Autodesk Fusion 360 part; units mm, degrees
(part 5 of 11)
  spline S19 degree 5 poles (23.435, -47.1498) (23.4194, -47.1502) (23.3882, -47.1511) (23.3415, -47.1525) (23.2792, -47.1547) (23.2015, -47.1578) (23.1239, -47.1612) (23.0464, -47.1651) (22.9691, -47.1693) (22.8919, -47.1739) (22.8149, -47.179) (22.738, -47.1844) (22.6613, -47.1902) (22.5846, -47.1964) (22.5082, -47.2031) (22.4319, -47.2101) (22.3558, -47.2175) (22.2798, -47.2253) (22.204, -47.2336) (22.1283, -47.2422) (22.0528, -47.2512) (21.9775, -47.2607) (21.9023, -47.2706) (21.8274, -47.2809) (21.7526, -47.2916) (21.6779, -47.3027) (21.6035, -47.3143) (21.5293, -47.3262) (21.4552, -47.3386) (21.3814, -47.3515) (21.3077, -47.3647) (21.2343, -47.3784) (21.161, -47.3926) (21.088, -47.4072) (21.0152, -47.4222) (20.9426, -47.4377) (20.8702, -47.4536) (20.7981, -47.47) (20.7261, -47.4868) (20.6545, -47.5041) (20.583, -47.5219) (20.5118, -47.5401) (20.4409, -47.5588) (20.3702, -47.5781) (20.2998, -47.5978) (20.2296, -47.6179) (20.1598, -47.6386) (20.0902, -47.6598) (20.0208, -47.6814) (19.9518, -47.7036) (19.8831, -47.7263) (19.8147, -47.7496) (19.7466, -47.7734) (19.679, -47.7979) (19.6116, -47.8229) (19.5446, -47.8485) (19.4779, -47.8745) (19.4115, -47.9011) (19.3455, -47.9282) (19.2798, -47.956) (19.2147, -47.9844) (19.15, -48.0138) (19.086, -48.044) (19.0226, -48.0751) (18.9598, -48.107) (18.8973, -48.1395) (18.8351, -48.1724) (18.7733, -48.2058) (18.7119, -48.2397) (18.6513, -48.2748) (18.5921, -48.3117) (18.5461, -48.3432) (18.5126, -48.3682) (18.4908, -48.3855) (18.48, -48.3944) knots -1 -1 -1 -1 -1 -1 -0.98571429 -0.97142857 -0.95714286 -0.94285714 -0.92857143 -0.91428571 -0.9 -0.88571429 -0.87142857 -0.85714286 -0.84285714 -0.82857143 -0.81428571 -0.8 -0.78571429 -0.77142857 -0.75714286 -0.74285714 -0.72857143 -0.71428571 -0.7 -0.68571429 -0.67142857 -0.65714286 -0.64285714 -0.62857143 -0.61428571 -0.6 -0.58571429 -0.57142857 -0.55714286 -0.54285714 -0.52857143 -0.51428571 -0.5 -0.48571429 -0.47142857 -0.45714286 -0.44285714 -0.42857143 -0.41428571 -0.4 -0.38571429 -0.37142857 -0.35714286 -0.34285714 -0.32857143 -0.31428571 -0.3 -0.28571429 -0.27142857 -0.25714286 -0.24285714 -0.22857143 -0.21428571 -0.2 -0.18571429 -0.17142857 -0.15714286 -0.14285714 -0.12857143 -0.11428571 -0.1 -0.08571429 -0.07142857 -0.05714286 -0.04285714 -0.02857143 -0.01428571 0 0 0 0 0 0
  line L19 (18.48, -48.3944) -> (17.8629, -48.8983)
  arc A39 (15.7015, -48.7555) -> (17.8629, -48.8983) centre (16.8587, -47.6688) ccw
  arc A40 (15.7015, -48.7555) -> (14.881, -47.9278) centre (0, -63.5) ccw
  arc A41 (14.757, -45.7652) -> (14.881, -47.9278) centre (15.9777, -46.7801) ccw
  line L20 (14.757, -45.7652) -> (15.2663, -45.1525)
  spline S20 degree 5 poles (15.2663, -45.1525) (15.2753, -45.1418) (15.2928, -45.1201) (15.3181, -45.0869) (15.35, -45.0412) (15.3874, -44.9822) (15.423, -44.922) (15.4575, -44.8609) (15.4914, -44.7993) (15.5248, -44.7375) (15.5579, -44.6753) (15.5903, -44.6127) (15.622, -44.5496) (15.6528, -44.4858) (15.6826, -44.4215) (15.7117, -44.3565) (15.74, -44.2911) (15.7677, -44.2253) (15.7948, -44.1592) (15.8215, -44.0927) (15.8476, -44.0259) (15.8733, -43.9588) (15.8983, -43.8913) (15.9227, -43.8235) (15.9466, -43.7553) (15.9699, -43.6868) (15.9927, -43.618) (16.0149, -43.5488) (16.0367, -43.4794) (16.058, -43.4097) (16.0788, -43.3398) (16.0991, -43.2695) (16.1189, -43.199) (16.1383, -43.1282) (16.1571, -43.0572) (16.1755, -42.9859) (16.1934, -42.9144) (16.2109, -42.8426) (16.2279, -42.7706) (16.2445, -42.6984) (16.2606, -42.6259) (16.2762, -42.5532) (16.2915, -42.4803) (16.3062, -42.4072) (16.3206, -42.3339) (16.3345, -42.2604) (16.348, -42.1866) (16.361, -42.1127) (16.3736, -42.0385) (16.3858, -41.9642) (16.3976, -41.8897) (16.409, -41.815) (16.4199, -41.7401) (16.4305, -41.6651) (16.4406, -41.5898) (16.4503, -41.5144) (16.4596, -41.4388) (16.4685, -41.3631) (16.477, -41.2872) (16.4851, -41.2111) (16.4927, -41.1349) (16.5, -41.0585) (16.5069, -40.9819) (16.5134, -40.9052) (16.5195, -40.8284) (16.5252, -40.7514) (16.5305, -40.6743) (16.5354, -40.597) (16.54, -40.5196) (16.5441, -40.442) (16.5478, -40.3643) (16.5505, -40.3021) (16.5524, -40.2553) (16.5535, -40.2241) (16.5541, -40.2085) knots 0 0 0 0 0 0 0.01428571 0.02857143 0.04285714 0.05714286 0.07142857 0.08571429 0.1 0.11428571 0.12857143 0.14285714 0.15714286 0.17142857 0.18571429 0.2 0.21428571 0.22857143 0.24285714 0.25714286 0.27142857 0.28571429 0.3 0.31428571 0.32857143 0.34285714 0.35714286 0.37142857 0.38571429 0.4 0.41428571 0.42857143 0.44285714 0.45714286 0.47142857 0.48571429 0.5 0.51428571 0.52857143 0.54285714 0.55714286 0.57142857 0.58571429 0.6 0.61428571 0.62857143 0.64285714 0.65714286 0.67142857 0.68571429 0.7 0.71428571 0.72857143 0.74285714 0.75714286 0.77142857 0.78571429 0.8 0.81428571 0.82857143 0.84285714 0.85714286 0.87142857 0.88571429 0.9 0.91428571 0.92857143 0.94285714 0.95714286 0.97142857 0.98571429 1 1 1 1 1 1
  arc A42 (16.5541, -40.2085) -> (15.3942, -39.4262) centre (0, -63.5) ccw
  spline S21 degree 5 poles (15.3942, -39.4262) (15.3799, -39.4325) (15.3514, -39.4453) (15.3088, -39.4645) (15.2521, -39.4903) (15.1815, -39.5229) (15.1111, -39.5558) (15.041, -39.589) (14.9712, -39.6225) (14.9017, -39.6563) (14.8324, -39.6905) (14.7635, -39.7249) (14.6948, -39.7596) (14.6264, -39.7947) (14.5583, -39.8301) (14.4905, -39.8658) (14.423, -39.9017) (14.3558, -39.9381) (14.2889, -39.9747) (14.2223, -40.0116) (14.156, -40.0489) (14.09, -40.0864) (14.0244, -40.1243) (13.9591, -40.1625) (13.8941, -40.201) (13.8294, -40.2399) (13.765, -40.279) (13.701, -40.3185) (13.6374, -40.3583) (13.574, -40.3984) (13.5111, -40.4389) (13.4485, -40.4796) (13.3862, -40.5207) (13.3243, -40.5621) (13.2628, -40.6039) (13.2016, -40.646) (13.1409, -40.6884) (13.0805, -40.7311) (13.0205, -40.7742) (12.9609, -40.8176) (12.9017, -40.8614) (12.8429, -40.9055) (12.7845, -40.9499) (12.7265, -40.9947) (12.669, -41.0398) (12.612, -41.0853) (12.5553, -41.1312) (12.4991, -41.1774) (12.4433, -41.2239) (12.388, -41.2708) (12.3332, -41.3181) (12.279, -41.3658) (12.2252, -41.4138) (12.172, -41.4623) (12.1194, -41.5112) (12.0673, -41.5605) (12.0156, -41.6101) (11.9645, -41.66) (11.9139, -41.7104) (11.8638, -41.7611) (11.8145, -41.8124) (11.766, -41.8642) (11.7184, -41.9166) (11.6718, -41.9696) (11.6259, -42.0231) (11.5806, -42.0771) (11.5358, -42.1313) (11.4914, -42.1858) (11.4477, -42.2406) (11.4052, -42.2962) (11.3645, -42.3529) (11.3341, -42.3996) (11.3128, -42.4356) (11.2992, -42.4599) (11.2926, -42.4722) knots -1 -1 -1 -1 -1 -1 -0.98571429 -0.97142857 -0.95714286 -0.94285714 -0.92857143 -0.91428571 -0.9 -0.88571429 -0.87142857 -0.85714286 -0.84285714 -0.82857143 -0.81428571 -0.8 -0.78571429 -0.77142857 -0.75714286 -0.74285714 -0.72857143 -0.71428571 -0.7 -0.68571429 -0.67142857 -0.65714286 -0.64285714 -0.62857143 -0.61428571 -0.6 -0.58571429 -0.57142857 -0.55714286 -0.54285714 -0.52857143 -0.51428571 -0.5 -0.48571429 -0.47142857 -0.45714286 -0.44285714 -0.42857143 -0.41428571 -0.4 -0.38571429 -0.37142857 -0.35714286 -0.34285714 -0.32857143 -0.31428571 -0.3 -0.28571429 -0.27142857 -0.25714286 -0.24285714 -0.22857143 -0.21428571 -0.2 -0.18571429 -0.17142857 -0.15714286 -0.14285714 -0.12857143 -0.11428571 -0.1 -0.08571429 -0.07142857 -0.05714286 -0.04285714 -0.02857143 -0.01428571 0 0 0 0 0 0
  line L21 (11.2926, -42.4722) -> (10.9153, -43.174)
  arc A43 (8.8638, -43.8692) -> (10.9153, -43.174) centre (9.5171, -42.4223) ccw
  arc A44 (8.8638, -43.8692) -> (7.789, -43.4184) centre (0, -63.5) ccw
  arc A45 (6.8469, -41.4679) -> (7.789, -43.4184) centre (8.3631, -41.9384) ccw
  line L22 (6.8469, -41.4679) -> (7.083, -40.707)
  spline S22 degree 5 poles (7.083, -40.707) (7.0871, -40.6936) (7.095, -40.6669) (7.1057, -40.6265) (7.1177, -40.5721) (7.1297, -40.5033) (7.1395, -40.434) (7.148, -40.3644) (7.1557, -40.2946) (7.163, -40.2246) (7.1697, -40.1545) (7.1757, -40.0843) (7.1808, -40.0138) (7.1849, -39.9431) (7.1878, -39.8722) (7.1898, -39.8012) (7.1909, -39.7299) (7.1913, -39.6585) (7.1911, -39.587) (7.1903, -39.5154) (7.1889, -39.4437) (7.1869, -39.3719) (7.1842, -39.3) (7.1808, -39.2279) (7.1768, -39.1558) (7.1721, -39.0836) (7.1668, -39.0113) (7.1609, -38.9389) (7.1544, -38.8664) (7.1474, -38.7939) (7.1399, -38.7213) (7.1318, -38.6486) (7.1231, -38.5759) (7.1139, -38.5031) (7.1041, -38.4303) (7.0938, -38.3574) (7.083, -38.2844) (7.0717, -38.2114) (7.0598, -38.1384) (7.0475, -38.0653) (7.0346, -37.9922) (7.0213, -37.9191) (7.0075, -37.8459) (6.9931, -37.7727) (6.9783, -37.6994) (6.963, -37.6262) (6.9473, -37.5529) (6.931, -37.4796) (6.9143, -37.4063) (6.8972, -37.3329) (6.8795, -37.2596) (6.8614, -37.1862) (6.8429, -37.1129) (6.8239, -37.0395) (6.8045, -36.9661) (6.7846, -36.8927) (6.7642, -36.8193) (6.7435, -36.746) (6.7223, -36.6726) (6.7006, -36.5992) (6.6785, -36.5258) (6.656, -36.4525) (6.6331, -36.3791) (6.6098, -36.3058) (6.586, -36.2324) (6.5618, -36.1591) (6.5372, -36.0858) (6.5121, -36.0125) (6.4867, -35.9393) (6.4608, -35.8661) (6.4346, -35.7929) (6.4132, -35.7343) (6.3971, -35.6904) (6.3862, -35.6611) (6.3807, -35.6465) knots 0 0 0 0 0 0 0.01428571 0.02857143 0.04285714 0.05714286 0.07142857 0.08571429 0.1 0.11428571 0.12857143 0.14285714 0.15714286 0.17142857 0.18571429 0.2 0.21428571 0.22857143 0.24285714 0.25714286 0.27142857 0.28571429 0.3 0.31428571 0.32857143 0.34285714 0.35714286 0.37142857 0.38571429 0.4 0.41428571 0.42857143 0.44285714 0.45714286 0.47142857 0.48571429 0.5 0.51428571 0.52857143 0.54285714 0.55714286 0.57142857 0.58571429 0.6 0.61428571 0.62857143 0.64285714 0.65714286 0.67142857 0.68571429 0.7 0.71428571 0.72857143 0.74285714 0.75714286 0.77142857 0.78571429 0.8 0.81428571 0.82857143 0.84285714 0.85714286 0.87142857 0.88571429 0.9 0.91428571 0.92857143 0.94285714 0.95714286 0.97142857 0.98571429 1 1 1 1 1 1
  arc A46 (6.3807, -35.6465) -> (5.0097, -35.3676) centre (0, -63.5) ccw
  spline S23 degree 5 poles (5.0097, -35.3676) (4.999, -35.3789) (4.9776, -35.4016) (4.9455, -35.4357) (4.903, -35.4812) (4.8502, -35.5384) (4.7978, -35.5957) (4.7457, -35.6532) (4.6941, -35.7108) (4.6428, -35.7687) (4.5919, -35.8267) (4.5413, -35.8849) (4.4912, -35.9433) (4.4414, -36.0019) (4.392, -36.0606) (4.343, -36.1195) (4.2944, -36.1786) (4.2462, -36.2379) (4.1984, -36.2973) (4.1511, -36.3569) (4.1041, -36.4167) (4.0575, -36.4767) (4.0114, -36.5368) (3.9656, -36.5971) (3.9203, -36.6575) (3.8754, -36.7182) (3.831, -36.779) (3.7869, -36.8399) (3.7433, -36.9011) (3.7002, -36.9624) (3.6575, -37.0238) (3.6152, -37.0854) (3.5735, -37.1472) (3.5321, -37.2092) (3.4913, -37.2713) (3.4509, -37.3336) (3.411, -37.396) (3.3715, -37.4586) (3.3326, -37.5214) (3.2941, -37.5843) (3.2561, -37.6474) (3.2187, -37.7106) (3.1818, -37.774) (3.1454, -37.8376) (3.1095, -37.9013) (3.0742, -37.9652) (3.0394, -38.0292) (3.0052, -38.0934) (2.9715, -38.1577) (2.9383, -38.2222) (2.9058, -38.2869) (2.8739, -38.3517) (2.8426, -38.4167) (2.812, -38.4818) (2.7821, -38.5471) (2.7528, -38.6126) (2.7241, -38.6782) (2.696, -38.7439) (2.6684, -38.8098) (2.6416, -38.8758) (2.6157, -38.942) (2.5907, -39.0084) (2.5668, -39.0751) (2.544, -39.1419) (2.5221, -39.2089) (2.5009, -39.2761) (2.4802, -39.3433) (2.4601, -39.4106) (2.4407, -39.478) (2.4226, -39.5457) (2.4068, -39.6136) (2.3966, -39.6684) (2.3906, -39.7098) (2.3874, -39.7375) (2.386, -39.7514) knots -1 -1 -1 -1 -1 -1 -0.98571429 -0.97142857 -0.95714286 -0.94285714 -0.92857143 -0.91428571 -0.9 -0.88571429 -0.87142857 -0.85714286 -0.84285714 -0.82857143 -0.81428571 -0.8 -0.78571429 -0.77142857 -0.75714286 -0.74285714 -0.72857143 -0.71428571 -0.7 -0.68571429 -0.67142857 -0.65714286 -0.64285714 -0.62857143 -0.61428571 -0.6 -0.58571429 -0.57142857 -0.55714286 -0.54285714 -0.52857143 -0.51428571 -0.5 -0.48571429 -0.47142857 -0.45714286 -0.44285714 -0.42857143 -0.41428571 -0.4 -0.38571429 -0.37142857 -0.35714286 -0.34285714 -0.32857143 -0.31428571 -0.3 -0.28571429 -0.27142857 -0.25714286 -0.24285714 -0.22857143 -0.21428571 -0.2 -0.18571429 -0.17142857 -0.15714286 -0.14285714 -0.12857143 -0.11428571 -0.1 -0.08571429 -0.07142857 -0.05714286 -0.04285714 -0.02857143 -0.01428571 0 0 0 0 0 0
  line L23 (2.386, -39.7514) -> (2.306, -40.5441)
  arc A47 (0.6767, -41.9714) -> (2.306, -40.5441) centre (0.7266, -40.3847) ccw
  arc A48 (0.6767, -41.9714) -> (-0.4888, -41.9663) centre (0, -63.5) ccw
  arc A49 (-2.1056, -40.5248) -> (-0.4888, -41.9663) centre (-0.5248, -40.3793) ccw
  line L24 (-2.1056, -40.5248) -> (-2.1787, -39.7315)
  spline S24 degree 5 poles (-2.1787, -39.7315) (-2.18, -39.7176) (-2.1829, -39.6898) (-2.1885, -39.6484) (-2.1983, -39.5936) (-2.2135, -39.5254) (-2.231, -39.4577) (-2.2498, -39.3901) (-2.2693, -39.3226) (-2.2894, -39.2552) (-2.31, -39.1878) (-2.3313, -39.1206) (-2.3535, -39.0536) (-2.3769, -38.9868) (-2.4013, -38.9201) (-2.4266, -38.8537) (-2.4529, -38.7874) (-2.4798, -38.7213) (-2.5074, -38.6553) (-2.5355, -38.5895) (-2.5643, -38.5238) (-2.5936, -38.4582) (-2.6236, -38.3928) (-2.6543, -38.3276) (-2.6856, -38.2625) (-2.7176, -38.1975) (-2.7502, -38.1328) (-2.7833, -38.0681) (-2.817, -38.0036) (-2.8513, -37.9393) (-2.886, -37.8751) (-2.9213, -37.8111) (-2.9572, -37.7472) (-2.9935, -37.6835) (-3.0304, -37.6199) (-3.0678, -37.5565) (-3.1057, -37.4933) (-3.1441, -37.4302) (-3.183, -37.3672) (-3.2224, -37.3045) (-3.2622, -37.2418) (-3.3026, -37.1794) (-3.3433, -37.117) (-3.3846, -37.0549) (-3.4263, -36.9929) (-3.4685, -36.9311) (-3.5111, -36.8694) (-3.5541, -36.8079) (-3.5976, -36.7465) (-3.6416, -36.6854) (-3.6859, -36.6243) (-3.7307, -36.5635) (-3.7759, -36.5028) (-3.8215, -36.4423) (-3.8676, -36.3819) (-3.914, -36.3217) (-3.9609, -36.2617) (-4.0082, -36.2019) (-4.0559, -36.1422) (-4.1039, -36.0827) (-4.1524, -36.0233) (-4.2013, -35.9642) (-4.2505, -35.9052) (-4.3002, -35.8464) (-4.3502, -35.7877) (-4.4006, -35.7292) (-4.4514, -35.6709) (-4.5026, -35.6128) (-4.5541, -35.5549) (-4.606, -35.4971) (-4.6583, -35.4395) (-4.7004, -35.3936) (-4.7322, -35.3592) (-4.7534, -35.3364) (-4.764, -35.3249) knots 0 0 0 0 0 0 0.01428571 0.02857143 0.04285714 0.05714286 0.07142857 0.08571429 0.1 0.11428571 0.12857143 0.14285714 0.15714286 0.17142857 0.18571429 0.2 0.21428571 0.22857143 0.24285714 0.25714286 0.27142857 0.28571429 0.3 0.31428571 0.32857143 0.34285714 0.35714286 0.37142857 0.38571429 0.4 0.41428571 0.42857143 0.44285714 0.45714286 0.47142857 0.48571429 0.5 0.51428571 0.52857143 0.54285714 0.55714286 0.57142857 0.58571429 0.6 0.61428571 0.62857143 0.64285714 0.65714286 0.67142857 0.68571429 0.7 0.71428571 0.72857143 0.74285714 0.75714286 0.77142857 0.78571429 0.8 0.81428571 0.82857143 0.84285714 0.85714286 0.87142857 0.88571429 0.9 0.91428571 0.92857143 0.94285714 0.95714286 0.97142857 0.98571429 1 1 1 1 1 1
  arc A50 (-4.764, -35.3249) -> (-6.1374, -35.5919) centre (0, -63.5) ccw
  spline S25 degree 5 poles (-6.1374, -35.5919) (-6.143, -35.6065) (-6.1541, -35.6356) (-6.1707, -35.6794) (-6.1925, -35.7378) (-6.2194, -35.8107) (-6.2459, -35.8837) (-6.272, -35.9568) (-6.2977, -36.0298) (-6.3229, -36.1029) (-6.3478, -36.176) (-6.3722, -36.2491) (-6.3962, -36.3222) (-6.4198, -36.3954) (-6.4429, -36.4686) (-6.4656, -36.5417) (-6.4879, -36.6149) (-6.5097, -36.6881) (-6.5312, -36.7613) (-6.5521, -36.8345) (-6.5727, -36.9077) (-6.5927, -36.9809) (-6.6124, -37.0542) (-6.6316, -37.1274) (-6.6503, -37.2006) (-6.6686, -37.2738) (-6.6864, -37.3469) (-6.7037, -37.4201) (-6.7206, -37.4933) (-6.737, -37.5664) (-6.7529, -37.6395) (-6.7684, -37.7126) (-6.7833, -37.7857) (-6.7978, -37.8588) (-6.8118, -37.9318) (-6.8253, -38.0048) (-6.8383, -38.0777) (-6.8507, -38.1507) (-6.8627, -38.2236) (-6.8742, -38.2964) (-6.8851, -38.3692) (-6.8955, -38.442) (-6.9053, -38.5147) (-6.9146, -38.5873) (-6.9234, -38.6599) (-6.9316, -38.7324) (-6.9392, -38.8049) (-6.9463, -38.8773) (-6.9528, -38.9497) (-6.9587, -39.0219) (-6.9641, -39.0941) (-6.9687, -39.1662) (-6.9727, -39.2382) (-6.9761, -39.3101) (-6.9787, -39.3819) (-6.9807, -39.4536) (-6.9822, -39.5251) (-6.983, -39.5966) (-6.9832, -39.668) (-6.9827, -39.7393) (-6.9814, -39.8104) (-6.979, -39.8813) (-6.9756, -39.952) (-6.9711, -40.0225) (-6.9657, -40.0928) (-6.9596, -40.163) (-6.9529, -40.233) (-6.9458, -40.3029) (-6.9379, -40.3726) (-6.9287, -40.442) (-6.9173, -40.5108) (-6.9058, -40.5654) (-6.8955, -40.6059) (-6.8878, -40.6327) (-6.8838, -40.646) knots -1 -1 -1 -1 -1 -1 -0.98571429 -0.97142857 -0.95714286 -0.94285714 -0.92857143 -0.91428571 -0.9 -0.88571429 -0.87142857 -0.85714286 -0.84285714 -0.82857143 -0.81428571 -0.8 -0.78571429 -0.77142857 -0.75714286 -0.74285714 -0.72857143 -0.71428571 -0.7 -0.68571429 -0.67142857 -0.65714286 -0.64285714 -0.62857143 -0.61428571 -0.6 -0.58571429 -0.57142857 -0.55714286 -0.54285714 -0.52857143 -0.51428571 -0.5 -0.48571429 -0.47142857 -0.45714286 -0.44285714 -0.42857143 -0.41428571 -0.4 -0.38571429 -0.37142857 -0.35714286 -0.34285714 -0.32857143 -0.31428571 -0.3 -0.28571429 -0.27142857 -0.25714286 -0.24285714 -0.22857143 -0.21428571 -0.2 -0.18571429 -0.17142857 -0.15714286 -0.14285714 -0.12857143 -0.11428571 -0.1 -0.08571429 -0.07142857 -0.05714286 -0.04285714 -0.02857143 -0.01428571 0 0 0 0 0 0
  line L25 (-6.8838, -40.646) -> (-6.6544, -41.409)
  arc A51 (-7.6135, -43.3512) -> (-6.6544, -41.409) centre (-8.1746, -41.8662) ccw
  arc A52 (-7.6135, -43.3512) -> (-8.6921, -43.7925) centre (0, -63.5) ccw
  arc A53 (-10.7376, -43.0795) -> (-8.6921, -43.7925) centre (-9.3328, -42.3401) ccw
  line L26 (-10.7376, -43.0795) -> (-11.1087, -42.3745)
  spline S26 degree 5 poles (-11.1087, -42.3745) (-11.1152, -42.3621) (-11.1285, -42.3376) (-11.1495, -42.3015) (-11.1795, -42.2546) (-11.2197, -42.1975) (-11.2617, -42.1415) (-11.305, -42.0863) (-11.3489, -42.0314) (-11.3932, -41.9768) (-11.438, -41.9225) (-11.4834, -41.8686) (-11.5296, -41.8151) (-11.5767, -41.7623) (-11.6248, -41.7101) (-11.6737, -41.6584) (-11.7233, -41.6072) (-11.7734, -41.5565) (-11.8242, -41.5061) (-11.8754, -41.456) (-11.9271, -41.4063) (-11.9793, -41.3569) (-12.032, -41.308) (-12.0853, -41.2595) (-12.1392, -41.2113) (-12.1936, -41.1636) (-12.2485, -41.1162) (-12.3038, -41.0692) (-12.3596, -41.0225) (-12.4159, -40.9761) (-12.4726, -40.9301) (-12.5297, -40.8845) (-12.5872, -40.8392) (-12.6452, -40.7942) (-12.7036, -40.7496) (-12.7624, -40.7054) (-12.8217, -40.6614) (-12.8813, -40.6178) (-12.9413, -40.5746) (-13.0017, -40.5316) (-13.0625, -40.489) (-13.1236, -40.4467) (-13.1852, -40.4048) (-13.2471, -40.3631) (-13.3093, -40.3218) (-13.3719, -40.2808) (-13.4349, -40.2402) (-13.4982, -40.1998) (-13.5619, -40.1598) (-13.6259, -40.1201) (-13.6902, -40.0807) (-13.7549, -40.0416) (-13.8199, -40.0028) (-13.8852, -39.9644) (-13.9508, -39.9262) (-14.0168, -39.8884) (-14.083, -39.8509) (-14.1496, -39.8137) (-14.2165, -39.7768) (-14.2837, -39.7402) (-14.3512, -39.7039) (-14.419, -39.668) (-14.4871, -39.6323) (-14.5554, -39.597) (-14.6241, -39.5619) (-14.693, -39.5272) (-14.7623, -39.4928) (-14.8318, -39.4587) (-14.9016, -39.4248) (-14.9716, -39.3913) (-15.042, -39.3582) (-15.0985, -39.3318) (-15.141, -39.3122) (-15.1693, -39.2992) (-15.1835, -39.2928) knots 0 0 0 0 0 0 0.01428571 0.02857143 0.04285714 0.05714286 0.07142857 0.08571429 0.1 0.11428571 0.12857143 0.14285714 0.15714286 0.17142857 0.18571429 0.2 0.21428571 0.22857143 0.24285714 0.25714286 0.27142857 0.28571429 0.3 0.31428571 0.32857143 0.34285714 0.35714286 0.37142857 0.38571429 0.4 0.41428571 0.42857143 0.44285714 0.45714286 0.47142857 0.48571429 0.5 0.51428571 0.52857143 0.54285714 0.55714286 0.57142857 0.58571429 0.6 0.61428571 0.62857143 0.64285714 0.65714286 0.67142857 0.68571429 0.7 0.71428571 0.72857143 0.74285714 0.75714286 0.77142857 0.78571429 0.8 0.81428571 0.82857143 0.84285714 0.85714286 0.87142857 0.88571429 0.9 0.91428571 0.92857143 0.94285714 0.95714286 0.97142857 0.98571429 1 1 1 1 1 1
  arc A54 (-15.1835, -39.2928) -> (-16.3502, -40.065) centre (0, -63.5) ccw
  spline S27 degree 5 poles (-16.3502, -40.065) (-16.3498, -40.0806) (-16.3489, -40.1118) (-16.3475, -40.1585) (-16.3453, -40.2208) (-16.3422, -40.2985) (-16.3388, -40.3761) (-16.3349, -40.4536) (-16.3307, -40.5309) (-16.3261, -40.6081) (-16.321, -40.6851) (-16.3156, -40.762) (-16.3098, -40.8387) (-16.3036, -40.9154) (-16.2969, -40.9918) (-16.2899, -41.0681) (-16.2825, -41.1442) (-16.2747, -41.2202) (-16.2664, -41.296) (-16.2578, -41.3717) (-16.2488, -41.4472) (-16.2393, -41.5225) (-16.2294, -41.5977) (-16.2191, -41.6726) (-16.2084, -41.7474) (-16.1973, -41.8221) (-16.1857, -41.8965) (-16.1738, -41.9707) (-16.1614, -42.0448) (-16.1485, -42.1186) (-16.1353, -42.1923) (-16.1216, -42.2657) (-16.1074, -42.339) (-16.0928, -42.412) (-16.0778, -42.4848) (-16.0623, -42.5574) (-16.0464, -42.6298) (-16.03, -42.7019) (-16.0132, -42.7739) (-15.9959, -42.8455) (-15.9781, -42.917) (-15.9599, -42.9882) (-15.9412, -43.0591) (-15.9219, -43.1298) (-15.9022, -43.2002) (-15.8821, -43.2704) (-15.8614, -43.3402) (-15.8402, -43.4098) (-15.8186, -43.4792) (-15.7964, -43.5482) (-15.7737, -43.6169) (-15.7504, -43.6853) (-15.7266, -43.7534) (-15.7021, -43.821) (-15.6771, -43.8884) (-15.6515, -43.9554) (-15.6255, -44.0221) (-15.5989, -44.0885) (-15.5718, -44.1545) (-15.544, -44.2202) (-15.5156, -44.2853) (-15.4862, -44.35) (-15.456, -44.414) (-15.4249, -44.4774) (-15.393, -44.5402) (-15.3605, -44.6027) (-15.3276, -44.6649) (-15.2942, -44.7267) (-15.2603, -44.7881) (-15.2252, -44.8487) (-15.1883, -44.9079) (-15.1568, -44.9539) (-15.1318, -44.9874) (-15.1145, -45.0092) (-15.1056, -45.02) knots -1 -1 -1 -1 -1 -1 -0.98571429 -0.97142857 -0.95714286 -0.94285714 -0.92857143 -0.91428571 -0.9 -0.88571429 -0.87142857 -0.85714286 -0.84285714 -0.82857143 -0.81428571 -0.8 -0.78571429 -0.77142857 -0.75714286 -0.74285714 -0.72857143 -0.71428571 -0.7 -0.68571429 -0.67142857 -0.65714286 -0.64285714 -0.62857143 -0.61428571 -0.6 -0.58571429 -0.57142857 -0.55714286 -0.54285714 -0.52857143 -0.51428571 -0.5 -0.48571429 -0.47142857 -0.45714286 -0.44285714 -0.42857143 -0.41428571 -0.4 -0.38571429 -0.37142857 -0.35714286 -0.34285714 -0.32857143 -0.31428571 -0.3 -0.28571429 -0.27142857 -0.25714286 -0.24285714 -0.22857143 -0.21428571 -0.2 -0.18571429 -0.17142857 -0.15714286 -0.14285714 -0.12857143 -0.11428571 -0.1 -0.08571429 -0.07142857 -0.05714286 -0.04285714 -0.02857143 -0.01428571 0 0 0 0 0 0
  line L27 (-15.1056, -45.02) -> (-14.6017, -45.6371)
  arc A55 (-14.7445, -47.7985) -> (-14.6017, -45.6371) centre (-15.8312, -46.6413) ccw
  arc A56 (-14.7445, -47.7985) -> (-15.5722, -48.619) centre (0, -63.5) ccw
  arc A57 (-17.7348, -48.743) -> (-15.5722, -48.619) centre (-16.7199, -47.5223) ccw
  line L28 (-17.7348, -48.743) -> (-18.3475, -48.2337)
  spline S28 degree 5 poles (-18.3475, -48.2337) (-18.3582, -48.2247) (-18.3799, -48.2072) (-18.4131, -48.1819) (-18.4588, -48.15) (-18.5178, -48.1126) (-18.578, -48.077) (-18.6391, -48.0425) (-18.7007, -48.0086) (-18.7625, -47.9752) (-18.8247, -47.9421) (-18.8873, -47.9097) (-18.9504, -47.878) (-19.0142, -47.8472) (-19.0785, -47.8174) (-19.1435, -47.7883) (-19.2089, -47.76) (-19.2747, -47.7323) (-19.3408, -47.7052) (-19.4073, -47.6785) (-19.4741, -47.6524) (-19.5412, -47.6268) (-19.6087, -47.6017) (-19.6765, -47.5773) (-19.7447, -47.5534) (-19.8132, -47.5301) (-19.882, -47.5073) (-19.9512, -47.4851) (-20.0206, -47.4633) (-20.0903, -47.442) (-20.1602, -47.4212) (-20.2305, -47.4009) (-20.301, -47.3811) (-20.3718, -47.3617) (-20.4428, -47.3429) (-20.5141, -47.3245) (-20.5856, -47.3066) (-20.6574, -47.2891) (-20.7294, -47.2721) (-20.8016, -47.2555) (-20.8741, -47.2394) (-20.9468, -47.2238) (-21.0197, -47.2085) (-21.0928, -47.1938) (-21.1661, -47.1794) (-21.2396, -47.1655) (-21.3134, -47.152) (-21.3873, -47.139) (-21.4615, -47.1264) (-21.5358, -47.1142) (-21.6103, -47.1024) (-21.685, -47.091) (-21.7599, -47.0801) (-21.8349, -47.0695) (-21.9102, -47.0594) (-21.9856, -47.0497) (-22.0612, -47.0404) (-22.1369, -47.0315) (-22.2128, -47.023) (-22.2889, -47.0149) (-22.3651, -47.0073) (-22.4415, -47) (-22.5181, -46.9931) (-22.5948, -46.9866) (-22.6716, -46.9805) (-22.7486, -46.9748) (-22.8257, -46.9695) (-22.903, -46.9646) (-22.9804, -46.96) (-23.058, -46.9559) (-23.1357, -46.9522) (-23.1979, -46.9495) (-23.2447, -46.9476) (-23.2759, -46.9465) (-23.2915, -46.9459) knots 0 0 0 0 0 0 0.01428571 0.02857143 0.04285714 0.05714286 0.07142857 0.08571429 0.1 0.11428571 0.12857143 0.14285714 0.15714286 0.17142857 0.18571429 0.2 0.21428571 0.22857143 0.24285714 0.25714286 0.27142857 0.28571429 0.3 0.31428571 0.32857143 0.34285714 0.35714286 0.37142857 0.38571429 0.4 0.41428571 0.42857143 0.44285714 0.45714286 0.47142857 0.48571429 0.5 0.51428571 0.52857143 0.54285714 0.55714286 0.57142857 0.58571429 0.6 0.61428571 0.62857143 0.64285714 0.65714286 0.67142857 0.68571429 0.7 0.71428571 0.72857143 0.74285714 0.75714286 0.77142857 0.78571429 0.8 0.81428571 0.82857143 0.84285714 0.85714286 0.87142857 0.88571429 0.9 0.91428571 0.92857143 0.94285714 0.95714286 0.97142857 0.98571429 1 1 1 1 1 1
  arc A58 (-23.2915, -46.9459) -> (-24.0738, -48.1058) centre (0, -63.5) ccw
  spline S29 degree 5 poles (-24.0738, -48.1058) (-24.0675, -48.1201) (-24.0547, -48.1486) (-24.0355, -48.1912) (-24.0097, -48.2479) (-23.9771, -48.3185) (-23.9442, -48.3889) (-23.911, -48.459) (-23.8775, -48.5288) (-23.8437, -48.5983) (-23.8095, -48.6676) (-23.7751, -48.7365) (-23.7404, -48.8052) (-23.7053, -48.8736) (-23.6699, -48.9417) (-23.6342, -49.0095) (-23.5983, -49.077) (-23.5619, -49.1442) (-23.5253, -49.2111) (-23.4884, -49.2777) (-23.4511, -49.344) (-23.4136, -49.41) (-23.3757, -49.4756) (-23.3375, -49.5409) (-23.299, -49.6059) (-23.2601, -49.6706) (-23.221, -49.735) (-23.1815, -49.799) (-23.1417, -49.8626) (-23.1016, -49.926) (-23.0611, -49.9889) (-23.0204, -50.0515) (-22.9793, -50.1138) (-22.9379, -50.1757) (-22.8961, -50.2372) (-22.854, -50.2984) (-22.8116, -50.3591) (-22.7689, -50.4195) (-22.7258, -50.4795) (-22.6824, -50.5391) (-22.6386, -50.5983) (-22.5945, -50.6571) (-22.5501, -50.7155) (-22.5053, -50.7735) (-22.4602, -50.831) (-22.4147, -50.888) (-22.3688, -50.9447) (-22.3226, -51.0009) (-22.2761, -51.0567) (-22.2292, -51.112) (-22.1819, -51.1668) (-22.1342, -51.221) (-22.0862, -51.2748) (-22.0377, -51.328) (-21.9888, -51.3806) (-21.9395, -51.4327) (-21.8899, -51.4844) (-21.84, -51.5355) (-21.7896, -51.5861) (-21.7389, -51.6362) (-21.6876, -51.6855) (-21.6358, -51.734) (-21.5834, -51.7816) (-21.5304, -51.8282) (-21.4769, -51.8741) (-21.4229, -51.9194) (-21.3687, -51.9642) (-21.3142, -52.0086) (-21.2594, -52.0523) (-21.2038, -52.0949) (-21.1471, -52.1355) (-21.1004, -52.1659) (-21.0644, -52.1872) (-21.0401, -52.2008) (-21.0278, -52.2074) knots -1 -1 -1 -1 -1 -1 -0.98571429 -0.97142857 -0.95714286 -0.94285714 -0.92857143 -0.91428571 -0.9 -0.88571429 -0.87142857 -0.85714286 -0.84285714 -0.82857143 -0.81428571 -0.8 -0.78571429 -0.77142857 -0.75714286 -0.74285714 -0.72857143 -0.71428571 -0.7 -0.68571429 -0.67142857 -0.65714286 -0.64285714 -0.62857143 -0.61428571 -0.6 -0.58571429 -0.57142857 -0.55714286 -0.54285714 -0.52857143 -0.51428571 -0.5 -0.48571429 -0.47142857 -0.45714286 -0.44285714 -0.42857143 -0.41428571 -0.4 -0.38571429 -0.37142857 -0.35714286 -0.34285714 -0.32857143 -0.31428571 -0.3 -0.28571429 -0.27142857 -0.25714286 -0.24285714 -0.22857143 -0.21428571 -0.2 -0.18571429 -0.17142857 -0.15714286 -0.14285714 -0.12857143 -0.11428571 -0.1 -0.08571429 -0.07142857 -0.05714286 -0.04285714 -0.02857143 -0.01428571 0 0 0 0 0 0
  line L29 (-21.0278, -52.2074) -> (-20.326, -52.5847)
  arc A59 (-19.6308, -54.6362) -> (-20.326, -52.5847) centre (-21.0777, -53.9829) ccw
  arc A60 (-19.6308, -54.6362) -> (-20.0816, -55.711) centre (0, -63.5) ccw
  arc A61 (-22.0321, -56.6531) -> (-20.0816, -55.711) centre (-21.5616, -55.1369) ccw
  line L30 (-22.0321, -56.6531) -> (-22.793, -56.417)
  spline S30 degree 5 poles (-22.793, -56.417) (-22.8063, -56.4129) (-22.8331, -56.405) (-22.8735, -56.3943) (-22.9279, -56.3823) (-22.9967, -56.3703) (-23.066, -56.3605) (-23.1356, -56.352) (-23.2054, -56.3443) (-23.2754, -56.337) (-23.3455, -56.3303) (-23.4157, -56.3243) (-23.4862, -56.3192) (-23.5569, -56.3151) (-23.6278, -56.3122) (-23.6988, -56.3102) (-23.7701, -56.3091) (-23.8415, -56.3087) (-23.913, -56.3089) (-23.9846, -56.3097) (-24.0563, -56.3111) (-24.1281, -56.3131) (-24.2, -56.3158) (-24.2721, -56.3192) (-24.3442, -56.3232) (-24.4164, -56.3279) (-24.4887, -56.3332) (-24.5611, -56.3391) (-24.6336, -56.3456) (-24.7061, -56.3526) (-24.7787, -56.3601) (-24.8514, -56.3682) (-24.9241, -56.3769) (-24.9969, -56.3861) (-25.0697, -56.3959) (-25.1426, -56.4062) (-25.2156, -56.417) (-25.2886, -56.4283) (-25.3616, -56.4402) (-25.4347, -56.4525) (-25.5078, -56.4654) (-25.5809, -56.4787) (-25.6541, -56.4925) (-25.7273, -56.5069) (-25.8006, -56.5217) (-25.8738, -56.537) (-25.9471, -56.5527) (-26.0204, -56.569) (-26.0937, -56.5857) (-26.1671, -56.6028) (-26.2404, -56.6205) (-26.3138, -56.6386) (-26.3871, -56.6571) (-26.4605, -56.6761) (-26.5339, -56.6955) (-26.6073, -56.7154) (-26.6807, -56.7358) (-26.754, -56.7565) (-26.8274, -56.7777) (-26.9008, -56.7994) (-26.9742, -56.8215) (-27.0475, -56.844) (-27.1209, -56.8669) (-27.1942, -56.8902) (-27.2676, -56.914) (-27.3409, -56.9382) (-27.4142, -56.9628) (-27.4875, -56.9879) (-27.5607, -57.0133) (-27.6339, -57.0392) (-27.7071, -57.0654) (-27.7657, -57.0868) (-27.8096, -57.1029) (-27.8389, -57.1138) (-27.8535, -57.1193) knots 0 0 0 0 0 0 0.01428571 0.02857143 0.04285714 0.05714286 0.07142857 0.08571429 0.1 0.11428571 0.12857143 0.14285714 0.15714286 0.17142857 0.18571429 0.2 0.21428571 0.22857143 0.24285714 0.25714286 0.27142857 0.28571429 0.3 0.31428571 0.32857143 0.34285714 0.35714286 0.37142857 0.38571429 0.4 0.41428571 0.42857143 0.44285714 0.45714286 0.47142857 0.48571429 0.5 0.51428571 0.52857143 0.54285714 0.55714286 0.57142857 0.58571429 0.6 0.61428571 0.62857143 0.64285714 0.65714286 0.67142857 0.68571429 0.7 0.71428571 0.72857143 0.74285714 0.75714286 0.77142857 0.78571429 0.8 0.81428571 0.82857143 0.84285714 0.85714286 0.87142857 0.88571429 0.9 0.91428571 0.92857143 0.94285714 0.95714286 0.97142857 0.98571429 1 1 1 1 1 1
  arc A62 (-27.8535, -57.1193) -> (-28.1324, -58.4903) centre (0, -63.5) ccw
  spline S31 degree 5 poles (-28.1324, -58.4903) (-28.1211, -58.501) (-28.0984, -58.5224) (-28.0643, -58.5545) (-28.0188, -58.597) (-27.9616, -58.6498) (-27.9043, -58.7022) (-27.8468, -58.7543) (-27.7892, -58.8059) (-27.7313, -58.8572) (-27.6733, -58.9081) (-27.6151, -58.9587) (-27.5567, -59.0088) (-27.4981, -59.0586) (-27.4394, -59.108) (-27.3805, -59.157) (-27.3214, -59.2056) (-27.2621, -59.2538) (-27.2027, -59.3016) (-27.1431, -59.3489) (-27.0833, -59.3959) (-27.0233, -59.4425) (-26.9632, -59.4886) (-26.9029, -59.5344) (-26.8425, -59.5797) (-26.7818, -59.6246) (-26.721, -59.669) (-26.6601, -59.7131) (-26.5989, -59.7567) (-26.5376, -59.7998) (-26.4762, -59.8425) (-26.4146, -59.8848) (-26.3528, -59.9265) (-26.2908, -59.9679) (-26.2287, -60.0087) (-26.1664, -60.0491) (-26.104, -60.089) (-26.0414, -60.1285) (-25.9786, -60.1674) (-25.9157, -60.2059) (-25.8526, -60.2439) (-25.7894, -60.2813) (-25.726, -60.3182) (-25.6624, -60.3546) (-25.5987, -60.3905) (-25.5348, -60.4258) (-25.4708, -60.4606) (-25.4066, -60.4948) (-25.3423, -60.5285) (-25.2778, -60.5617) (-25.2131, -60.5942) (-25.1483, -60.6261) (-25.0833, -60.6574) (-25.0182, -60.688) (-24.9529, -60.7179) (-24.8874, -60.7472) (-24.8218, -60.7759) (-24.7561, -60.804) (-24.6902, -60.8316) (-24.6242, -60.8584) (-24.558, -60.8843) (-24.4916, -60.9093) (-24.4249, -60.9332) (-24.3581, -60.956) (-24.2911, -60.9779) (-24.2239, -60.9991) (-24.1567, -61.0198) (-24.0894, -61.0399) (-24.022, -61.0593) (-23.9543, -61.0774) (-23.8864, -61.0932) (-23.8316, -61.1034) (-23.7902, -61.1094) (-23.7625, -61.1126) (-23.7486, -61.114) knots -1 -1 -1 -1 -1 -1 -0.98571429 -0.97142857 -0.95714286 -0.94285714 -0.92857143 -0.91428571 -0.9 -0.88571429 -0.87142857 -0.85714286 -0.84285714 -0.82857143 -0.81428571 -0.8 -0.78571429 -0.77142857 -0.75714286 -0.74285714 -0.72857143 -0.71428571 -0.7 -0.68571429 -0.67142857 -0.65714286 -0.64285714 -0.62857143 -0.61428571 -0.6 -0.58571429 -0.57142857 -0.55714286 -0.54285714 -0.52857143 -0.51428571 -0.5 -0.48571429 -0.47142857 -0.45714286 -0.44285714 -0.42857143 -0.41428571 -0.4 -0.38571429 -0.37142857 -0.35714286 -0.34285714 -0.32857143 -0.31428571 -0.3 -0.28571429 -0.27142857 -0.25714286 -0.24285714 -0.22857143 -0.21428571 -0.2 -0.18571429 -0.17142857 -0.15714286 -0.14285714 -0.12857143 -0.11428571 -0.1 -0.08571429 -0.07142857 -0.05714286 -0.04285714 -0.02857143 -0.01428571 0 0 0 0 0 0
  line L31 (-23.7486, -61.114) -> (-22.9559, -61.194)
  arc A63 (-21.5286, -62.8233) -> (-22.9559, -61.194) centre (-23.1153, -62.7734) ccw
  circle A64 centre (0, -63.5) radius 6.35
  circle A65 centre (0, -63.5) radius 6.35
  constraint concentric A0 A65
sketch "Sketch4" plane through (0, 0, 12.7) normal (0, 0, 1) x (-1, 0, 0)
  arc A0 (-7.9738, -97.7855) -> (-8.3356, -98.659) centre (0, -101.6) ccw
  arc A1 (-10.1257, -99.691) -> (-8.3356, -98.659) centre (-9.8326, -98.1307) ccw
  line L0 (-10.1257, -99.691) -> (-11.7277, -99.3901)
  spline S0 degree 5 poles (-11.7277, -99.3901) (-11.7394, -99.3879) (-11.7629, -99.3839) (-11.7983, -99.3793) (-11.8457, -99.3757) (-11.9054, -99.3747) (-11.9654, -99.3761) (-12.0256, -99.379) (-12.0858, -99.3828) (-12.1462, -99.3871) (-12.2066, -99.3921) (-12.267, -99.3979) (-12.3276, -99.4048) (-12.3882, -99.4131) (-12.4489, -99.4225) (-12.5096, -99.4331) (-12.5704, -99.4447) (-12.6312, -99.4571) (-12.692, -99.4702) (-12.7529, -99.4841) (-12.8137, -99.4986) (-12.8745, -99.5139) (-12.9353, -99.5301) (-12.9961, -99.547) (-13.0568, -99.5647) (-13.1176, -99.5832) (-13.1783, -99.6024) (-13.2389, -99.6223) (-13.2996, -99.6429) (-13.3602, -99.6642) (-13.4207, -99.6861) (-13.4812, -99.7086) (-13.5416, -99.7319) (-13.602, -99.7558) (-13.6622, -99.7804) (-13.7225, -99.8056) (-13.7826, -99.8314) (-13.8427, -99.8578) (-13.9026, -99.8849) (-13.9625, -99.9126) (-14.0223, -99.9409) (-14.082, -99.9697) (-14.1417, -99.9992) (-14.2012, -100.0293) (-14.2606, -100.0599) (-14.3199, -100.0911) (-14.379, -100.1229) (-14.4381, -100.1553) (-14.4971, -100.1882) (-14.5559, -100.2217) (-14.6146, -100.2558) (-14.6732, -100.2904) (-14.7316, -100.3255) (-14.7899, -100.3612) (-14.8481, -100.3974) (-14.9061, -100.4342) (-14.964, -100.4715) (-15.0217, -100.5093) (-15.0793, -100.5476) (-15.1368, -100.5865) (-15.194, -100.6259) (-15.2512, -100.6658) (-15.3081, -100.7062) (-15.3649, -100.7471) (-15.4216, -100.7885) (-15.478, -100.8304) (-15.5343, -100.8728) (-15.5904, -100.9157) (-15.6464, -100.9591) (-15.7021, -101.003) (-15.7577, -101.0474) (-15.802, -101.0833) (-15.8352, -101.1104) (-15.8572, -101.1286) (-15.8683, -101.1377) knots 0 0 0 0 0 0 0.01428571 0.02857143 0.04285714 0.05714286 0.07142857 0.08571429 0.1 0.11428571 0.12857143 0.14285714 0.15714286 0.17142857 0.18571429 0.2 0.21428571 0.22857143 0.24285714 0.25714286 0.27142857 0.28571429 0.3 0.31428571 0.32857143 0.34285714 0.35714286 0.37142857 0.38571429 0.4 0.41428571 0.42857143 0.44285714 0.45714286 0.47142857 0.48571429 0.5 0.51428571 0.52857143 0.54285714 0.55714286 0.57142857 0.58571429 0.6 0.61428571 0.62857143 0.64285714 0.65714286 0.67142857 0.68571429 0.7 0.71428571 0.72857143 0.74285714 0.75714286 0.77142857 0.78571429 0.8 0.81428571 0.82857143 0.84285714 0.85714286 0.87142857 0.88571429 0.9 0.91428571 0.92857143 0.94285714 0.95714286 0.97142857 0.98571429 1 1 1 1 1 1
  arc A2 (-15.8683, -101.1377) -> (-15.8683, -102.0623) centre (0, -101.6) ccw
  spline S1 degree 5 poles (-15.8683, -102.0623) (-15.8572, -102.0714) (-15.8352, -102.0896) (-15.802, -102.1167) (-15.7577, -102.1526) (-15.7021, -102.197) (-15.6464, -102.2409) (-15.5904, -102.2843) (-15.5343, -102.3272) (-15.478, -102.3696) (-15.4216, -102.4115) (-15.3649, -102.4529) (-15.3081, -102.4938) (-15.2512, -102.5342) (-15.194, -102.5741) (-15.1368, -102.6135) (-15.0793, -102.6524) (-15.0217, -102.6907) (-14.964, -102.7285) (-14.9061, -102.7658) (-14.8481, -102.8026) (-14.7899, -102.8388) (-14.7316, -102.8745) (-14.6732, -102.9096) (-14.6146, -102.9442) (-14.5559, -102.9783) (-14.4971, -103.0118) (-14.4381, -103.0447) (-14.379, -103.0771) (-14.3199, -103.1089) (-14.2606, -103.1401) (-14.2012, -103.1707) (-14.1417, -103.2008) (-14.082, -103.2303) (-14.0223, -103.2591) (-13.9625, -103.2874) (-13.9026, -103.3151) (-13.8427, -103.3422) (-13.7826, -103.3686) (-13.7225, -103.3944) (-13.6622, -103.4196) (-13.602, -103.4442) (-13.5416, -103.4681) (-13.4812, -103.4914) (-13.4207, -103.5139) (-13.3602, -103.5358) (-13.2996, -103.5571) (-13.2389, -103.5777) (-13.1783, -103.5976) (-13.1176, -103.6168) (-13.0568, -103.6353) (-12.9961, -103.653) (-12.9353, -103.6699) (-12.8745, -103.6861) (-12.8137, -103.7014) (-12.7529, -103.7159) (-12.692, -103.7298) (-12.6312, -103.7429) (-12.5704, -103.7553) (-12.5096, -103.7669) (-12.4489, -103.7775) (-12.3882, -103.7869) (-12.3276, -103.7952) (-12.267, -103.8021) (-12.2066, -103.8079) (-12.1462, -103.8129) (-12.0858, -103.8172) (-12.0256, -103.821) (-11.9654, -103.8239) (-11.9054, -103.8253) (-11.8457, -103.8243) (-11.7983, -103.8207) (-11.7629, -103.8161) (-11.7394, -103.8121) (-11.7277, -103.8099) knots -1 -1 -1 -1 -1 -1 -0.98571429 -0.97142857 -0.95714286 -0.94285714 -0.92857143 -0.91428571 -0.9 -0.88571429 -0.87142857 -0.85714286 -0.84285714 -0.82857143 -0.81428571 -0.8 -0.78571429 -0.77142857 -0.75714286 -0.74285714 -0.72857143 -0.71428571 -0.7 -0.68571429 -0.67142857 -0.65714286 -0.64285714 -0.62857143 -0.61428571 -0.6 -0.58571429 -0.57142857 -0.55714286 -0.54285714 -0.52857143 -0.51428571 -0.5 -0.48571429 -0.47142857 -0.45714286 -0.44285714 -0.42857143 -0.41428571 -0.4 -0.38571429 -0.37142857 -0.35714286 -0.34285714 -0.32857143 -0.31428571 -0.3 -0.28571429 -0.27142857 -0.25714286 -0.24285714 -0.22857143 -0.21428571 -0.2 -0.18571429 -0.17142857 -0.15714286 -0.14285714 -0.12857143 -0.11428571 -0.1 -0.08571429 -0.07142857 -0.05714286 -0.04285714 -0.02857143 -0.01428571 0 0 0 0 0 0
  line L1 (-11.7277, -103.8099) -> (-10.1257, -103.509)
  arc A3 (-8.3356, -104.541) -> (-10.1257, -103.509) centre (-9.8326, -105.0693) ccw
  arc A4 (-8.3356, -104.541) -> (-7.9738, -105.4145) centre (0, -101.6) ccw
  arc A5 (-8.5098, -107.41) -> (-7.9738, -105.4145) centre (-9.4058, -106.0996) ccw
  line L2 (-8.5098, -107.41) -> (-9.8554, -108.3301)
  spline S2 degree 5 poles (-9.8554, -108.3301) (-9.8652, -108.3368) (-9.8847, -108.3506) (-9.9129, -108.3724) (-9.949, -108.4034) (-9.992, -108.4449) (-10.0333, -108.4883) (-10.0738, -108.5329) (-10.1138, -108.5782) (-10.1534, -108.6239) (-10.1926, -108.6701) (-10.2312, -108.717) (-10.2691, -108.7647) (-10.3062, -108.8134) (-10.3424, -108.863) (-10.3779, -108.9134) (-10.4127, -108.9646) (-10.4469, -109.0164) (-10.4806, -109.0687) (-10.5138, -109.1214) (-10.5465, -109.1747) (-10.5787, -109.2286) (-10.6103, -109.2829) (-10.6413, -109.3379) (-10.6717, -109.3934) (-10.7016, -109.4494) (-10.731, -109.5059) (-10.7598, -109.5629) (-10.7881, -109.6204) (-10.8159, -109.6782) (-10.8432, -109.7365) (-10.87, -109.7952) (-10.8963, -109.8544) (-10.9221, -109.914) (-10.9473, -109.974) (-10.9721, -110.0344) (-10.9964, -110.0952) (-11.0201, -110.1564) (-11.0434, -110.2179) (-11.0662, -110.2798) (-11.0885, -110.3421) (-11.1103, -110.4047) (-11.1316, -110.4677) (-11.1524, -110.5311) (-11.1727, -110.5947) (-11.1926, -110.6587) (-11.212, -110.7231) (-11.2308, -110.7877) (-11.2492, -110.8527) (-11.2672, -110.918) (-11.2846, -110.9836) (-11.3015, -111.0494) (-11.318, -111.1156) (-11.334, -111.1821) (-11.3495, -111.2488) (-11.3646, -111.3158) (-11.3791, -111.3831) (-11.3932, -111.4507) (-11.4068, -111.5186) (-11.42, -111.5866) (-11.4326, -111.655) (-11.4448, -111.7236) (-11.4565, -111.7925) (-11.4678, -111.8615) (-11.4785, -111.9309) (-11.4888, -112.0004) (-11.4986, -112.0702) (-11.508, -112.1403) (-11.5168, -112.2105) (-11.5252, -112.2809) (-11.5331, -112.3516) (-11.5391, -112.4083) (-11.5434, -112.451) (-11.5461, -112.4794) (-11.5475, -112.4937) knots 0 0 0 0 0 0 0.01428571 0.02857143 0.04285714 0.05714286 0.07142857 0.08571429 0.1 0.11428571 0.12857143 0.14285714 0.15714286 0.17142857 0.18571429 0.2 0.21428571 0.22857143 0.24285714 0.25714286 0.27142857 0.28571429 0.3 0.31428571 0.32857143 0.34285714 0.35714286 0.37142857 0.38571429 0.4 0.41428571 0.42857143 0.44285714 0.45714286 0.47142857 0.48571429 0.5 0.51428571 0.52857143 0.54285714 0.55714286 0.57142857 0.58571429 0.6 0.61428571 0.62857143 0.64285714 0.65714286 0.67142857 0.68571429 0.7 0.71428571 0.72857143 0.74285714 0.75714286 0.77142857 0.78571429 0.8 0.81428571 0.82857143 0.84285714 0.85714286 0.87142857 0.88571429 0.9 0.91428571 0.92857143 0.94285714 0.95714286 0.97142857 0.98571429 1 1 1 1 1 1
  arc A6 (-11.5475, -112.4937) -> (-10.8937, -113.1475) centre (0, -101.6) ccw
  spline S3 degree 5 poles (-10.8937, -113.1475) (-10.8794, -113.1461) (-10.851, -113.1434) (-10.8083, -113.1391) (-10.7516, -113.1331) (-10.6809, -113.1252) (-10.6105, -113.1168) (-10.5403, -113.108) (-10.4702, -113.0986) (-10.4004, -113.0888) (-10.3309, -113.0785) (-10.2615, -113.0678) (-10.1925, -113.0565) (-10.1236, -113.0448) (-10.055, -113.0326) (-9.9866, -113.02) (-9.9186, -113.0068) (-9.8507, -112.9932) (-9.7831, -112.9791) (-9.7158, -112.9646) (-9.6488, -112.9495) (-9.5821, -112.934) (-9.5156, -112.918) (-9.4494, -112.9015) (-9.3836, -112.8846) (-9.318, -112.8672) (-9.2527, -112.8492) (-9.1877, -112.8308) (-9.1231, -112.812) (-9.0587, -112.7926) (-8.9947, -112.7727) (-8.9311, -112.7524) (-8.8677, -112.7316) (-8.8047, -112.7103) (-8.7421, -112.6885) (-8.6798, -112.6662) (-8.6179, -112.6434) (-8.5564, -112.6201) (-8.4952, -112.5964) (-8.4344, -112.5721) (-8.374, -112.5473) (-8.314, -112.5221) (-8.2544, -112.4963) (-8.1952, -112.47) (-8.1365, -112.4432) (-8.0782, -112.4159) (-8.0204, -112.3881) (-7.9629, -112.3598) (-7.9059, -112.331) (-7.8494, -112.3016) (-7.7934, -112.2717) (-7.7379, -112.2413) (-7.6829, -112.2103) (-7.6286, -112.1787) (-7.5747, -112.1465) (-7.5214, -112.1138) (-7.4687, -112.0806) (-7.4164, -112.0469) (-7.3646, -112.0127) (-7.3134, -111.9779) (-7.263, -111.9424) (-7.2134, -111.9062) (-7.1647, -111.8691) (-7.117, -111.8312) (-7.0701, -111.7926) (-7.0239, -111.7534) (-6.9782, -111.7138) (-6.9329, -111.6738) (-6.8883, -111.6333) (-6.8449, -111.592) (-6.8034, -111.549) (-6.7724, -111.5129) (-6.7506, -111.4847) (-6.7368, -111.4652) (-6.7301, -111.4554) knots -1 -1 -1 -1 -1 -1 -0.98571429 -0.97142857 -0.95714286 -0.94285714 -0.92857143 -0.91428571 -0.9 -0.88571429 -0.87142857 -0.85714286 -0.84285714 -0.82857143 -0.81428571 -0.8 -0.78571429 -0.77142857 -0.75714286 -0.74285714 -0.72857143 -0.71428571 -0.7 -0.68571429 -0.67142857 -0.65714286 -0.64285714 -0.62857143 -0.61428571 -0.6 -0.58571429 -0.57142857 -0.55714286 -0.54285714 -0.52857143 -0.51428571 -0.5 -0.48571429 -0.47142857 -0.45714286 -0.44285714 -0.42857143 -0.41428571 -0.4 -0.38571429 -0.37142857 -0.35714286 -0.34285714 -0.32857143 -0.31428571 -0.3 -0.28571429 -0.27142857 -0.25714286 -0.24285714 -0.22857143 -0.21428571 -0.2 -0.18571429 -0.17142857 -0.15714286 -0.14285714 -0.12857143 -0.11428571 -0.1 -0.08571429 -0.07142857 -0.05714286 -0.04285714 -0.02857143 -0.01428571 0 0 0 0 0 0
  line L3 (-6.7301, -111.4554) -> (-5.81, -110.1098)
  arc A7 (-3.8145, -109.5738) -> (-5.81, -110.1098) centre (-4.4996, -111.0058) ccw
  arc A8 (-3.8145, -109.5738) -> (-2.941, -109.9356) centre (0, -101.6) ccw
  arc A9 (-1.909, -111.7257) -> (-2.941, -109.9356) centre (-3.4693, -111.4326) ccw
  line L4 (-1.909, -111.7257) -> (-2.2099, -113.3277)
  spline S4 degree 5 poles (-2.2099, -113.3277) (-2.2121, -113.3394) (-2.2161, -113.3629) (-2.2207, -113.3983) (-2.2243, -113.4457) (-2.2253, -113.5054) (-2.2239, -113.5654) (-2.221, -113.6256) (-2.2172, -113.6858) (-2.2129, -113.7462) (-2.2079, -113.8066) (-2.2021, -113.867) (-2.1952, -113.9276) (-2.1869, -113.9882) (-2.1775, -114.0489) (-2.1669, -114.1096) (-2.1553, -114.1704) (-2.1429, -114.2312) (-2.1298, -114.292) (-2.1159, -114.3529) (-2.1014, -114.4137) (-2.0861, -114.4745) (-2.0699, -114.5353) (-2.053, -114.5961) (-2.0353, -114.6568) (-2.0168, -114.7176) (-1.9976, -114.7783) (-1.9777, -114.8389) (-1.9571, -114.8996) (-1.9358, -114.9602) (-1.9139, -115.0207) (-1.8914, -115.0812) (-1.8681, -115.1416) (-1.8442, -115.202) (-1.8196, -115.2622) (-1.7944, -115.3225) (-1.7686, -115.3826) (-1.7422, -115.4427) (-1.7151, -115.5026) (-1.6874, -115.5625) (-1.6591, -115.6223) (-1.6303, -115.682) (-1.6008, -115.7417) (-1.5707, -115.8012) (-1.5401, -115.8606) (-1.5089, -115.9199) (-1.4771, -115.979) (-1.4447, -116.0381) (-1.4118, -116.0971) (-1.3783, -116.1559) (-1.3442, -116.2146) (-1.3096, -116.2732) (-1.2745, -116.3316) (-1.2388, -116.3899) (-1.2026, -116.4481) (-1.1658, -116.5061) (-1.1285, -116.564) (-1.0907, -116.6217) (-1.0524, -116.6793) (-1.0135, -116.7368) (-0.9741, -116.794) (-0.9342, -116.8512) (-0.8938, -116.9081) (-0.8529, -116.9649) (-0.8115, -117.0216) (-0.7696, -117.078) (-0.7272, -117.1343) (-0.6843, -117.1904) (-0.6409, -117.2464) (-0.597, -117.3021) (-0.5526, -117.3577) (-0.5167, -117.402) (-0.4896, -117.4352) (-0.4714, -117.4572) (-0.4623, -117.4683) knots 0 0 0 0 0 0 0.01428571 0.02857143 0.04285714 0.05714286 0.07142857 0.08571429 0.1 0.11428571 0.12857143 0.14285714 0.15714286 0.17142857 0.18571429 0.2 0.21428571 0.22857143 0.24285714 0.25714286 0.27142857 0.28571429 0.3 0.31428571 0.32857143 0.34285714 0.35714286 0.37142857 0.38571429 0.4 0.41428571 0.42857143 0.44285714 0.45714286 0.47142857 0.48571429 0.5 0.51428571 0.52857143 0.54285714 0.55714286 0.57142857 0.58571429 0.6 0.61428571 0.62857143 0.64285714 0.65714286 0.67142857 0.68571429 0.7 0.71428571 0.72857143 0.74285714 0.75714286 0.77142857 0.78571429 0.8 0.81428571 0.82857143 0.84285714 0.85714286 0.87142857 0.88571429 0.9 0.91428571 0.92857143 0.94285714 0.95714286 0.97142857 0.98571429 1 1 1 1 1 1
  arc A10 (-0.4623, -117.4683) -> (0.4623, -117.4683) centre (0, -101.6) ccw
  spline S5 degree 5 poles (0.4623, -117.4683) (0.4714, -117.4572) (0.4896, -117.4352) (0.5167, -117.402) (0.5526, -117.3577) (0.597, -117.3021) (0.6409, -117.2464) (0.6843, -117.1904) (0.7272, -117.1343) (0.7696, -117.078) (0.8115, -117.0216) (0.8529, -116.9649) (0.8938, -116.9081) (0.9342, -116.8512) (0.9741, -116.794) (1.0135, -116.7368) (1.0524, -116.6793) (1.0907, -116.6217) (1.1285, -116.564) (1.1658, -116.5061) (1.2026, -116.4481) (1.2388, -116.3899) (1.2745, -116.3316) (1.3096, -116.2732) (1.3442, -116.2146) (1.3783, -116.1559) (1.4118, -116.0971) (1.4447, -116.0381) (1.4771, -115.979) (1.5089, -115.9199) (1.5401, -115.8606) (1.5707, -115.8012) (1.6008, -115.7417) (1.6303, -115.682) (1.6591, -115.6223) (1.6874, -115.5625) (1.7151, -115.5026) (1.7422, -115.4427) (1.7686, -115.3826) (1.7944, -115.3225) (1.8196, -115.2622) (1.8442, -115.202) (1.8681, -115.1416) (1.8914, -115.0812) (1.9139, -115.0207) (1.9358, -114.9602) (1.9571, -114.8996) (1.9777, -114.8389) (1.9976, -114.7783) (2.0168, -114.7176) (2.0353, -114.6568) (2.053, -114.5961) (2.0699, -114.5353) (2.0861, -114.4745) (2.1014, -114.4137) (2.1159, -114.3529) (2.1298, -114.292) (2.1429, -114.2312) (2.1553, -114.1704) (2.1669, -114.1096) (2.1775, -114.0489) (2.1869, -113.9882) (2.1952, -113.9276) (2.2021, -113.867) (2.2079, -113.8066) (2.2129, -113.7462) (2.2172, -113.6858) (2.221, -113.6256) (2.2239, -113.5654) (2.2253, -113.5054) (2.2243, -113.4457) (2.2207, -113.3983) (2.2161, -113.3629) (2.2121, -113.3394) (2.2099, -113.3277) knots -1 -1 -1 -1 -1 -1 -0.98571429 -0.97142857 -0.95714286 -0.94285714 -0.92857143 -0.91428571 -0.9 -0.88571429 -0.87142857 -0.85714286 -0.84285714 -0.82857143 -0.81428571 -0.8 -0.78571429 -0.77142857 -0.75714286 -0.74285714 -0.72857143 -0.71428571 -0.7 -0.68571429 -0.67142857 -0.65714286 -0.64285714 -0.62857143 -0.61428571 -0.6 -0.58571429 -0.57142857 -0.55714286 -0.54285714 -0.52857143 -0.51428571 -0.5 -0.48571429 -0.47142857 -0.45714286 -0.44285714 -0.42857143 -0.41428571 -0.4 -0.38571429 -0.37142857 -0.35714286 -0.34285714 -0.32857143 -0.31428571 -0.3 -0.28571429 -0.27142857 -0.25714286 -0.24285714 -0.22857143 -0.21428571 -0.2 -0.18571429 -0.17142857 -0.15714286 -0.14285714 -0.12857143 -0.11428571 -0.1 -0.08571429 -0.07142857 -0.05714286 -0.04285714 -0.02857143 -0.01428571 0 0 0 0 0 0
  line L5 (2.2099, -113.3277) -> (1.909, -111.7257)
  arc A11 (2.941, -109.9356) -> (1.909, -111.7257) centre (3.4693, -111.4326) ccw
  arc A12 (2.941, -109.9356) -> (3.8145, -109.5738) centre (0, -101.6) ccw
  arc A13 (5.81, -110.1098) -> (3.8145, -109.5738) centre (4.4996, -111.0058) ccw
  line L6 (5.81, -110.1098) -> (6.7301, -111.4554)